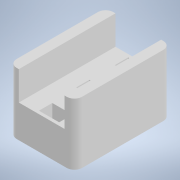
# Autodesk Inventor part: push-fit
Saved by Autodesk Inventor 2022 (Build 260153000, 153)
## iProperties
Created: 2024-10-14
Part Number: push-fit
Material: Типовые
Document SubType Name: Modeling
Designer: Andrey
Density: 1 g/cm^3
Appearance: По умолчанию
Author: Andrey
Autodesk Inventor part; units mm, degrees
ref_plane "YZ Plane" through (0, 0, 0) normal (1, 0, 0) x (0, 1, 0)
ref_plane "XZ Plane" through (0, 0, 0) normal (0, 1, 0) x (-1, 0, 0)
ref_plane "XY Plane" through (0, 0, 0) normal (0, 0, 1) x (1, 0, 0)
sketch "Эскиз1" plane through (0, 0, 0) normal (0, 1, 0) x (-1, 0, 0)
  line L0 (-2.9, 6.425) -> (2.9, 6.425)
  line L1 (2.9, 6.425) -> (2.9, -6.425)
  line L2 (2.9, -6.425) -> (-2.9, -6.425)
  line L3 (-2.9, -6.425) -> (-2.9, 6.425)
  line L4 (-2.9, 6.425) -> (2.9, -6.425) construction
  line L5 (2.9, 6.425) -> (-2.9, -6.425) construction
  line L6 (-3, 6.35) -> (3, 6.35)
  line L7 (3, 6.35) -> (3, -6.35)
  line L8 (3, -6.35) -> (-3, -6.35)
  line L9 (-3, -6.35) -> (-3, 6.35)
  line L10 (-3, 6.35) -> (3, -6.35) construction
  line L11 (3, 6.35) -> (-3, -6.35) construction
  line L12 (3, 6.35) -> (4.3, 6.35)
  line L13 (4.3, 6.35) -> (4.3, -6.35)
  line L14 (4.3, -6.35) -> (3, -6.35)
  line L15 (3, -6.35) -> (3, 6.35)
  line L16 (-3, 6.35) -> (-4.3, 6.35)
  line L17 (-4.3, 6.35) -> (-4.3, -6.35)
  line L18 (-4.3, -6.35) -> (-3, -6.35)
  line L19 (-3, -6.35) -> (-3, 6.35)
  point P0 (0, 0)
  dimension "d0" = 5.8
  dimension "d1" = 12.85
  dimension "d2" = 6
  dimension "d3" = 12.7
  dimension "d4" = 1.3
  dimension "d5" = 1.3
  constraints: 40 end point, 8 parallel, 4 horizontal, 4 midpoint, 4 perpendicular, 2 collinear
  measures "d0" distance of L1.end L2.end
  measures "d1" distance of L0.end L1.end
  measures "d2" distance of L7.end L8.end
  measures "d3" distance of L6.end L7.end
  measures "d4" distance of L13.end L14.end
  measures "d5" distance of L18.end L17.end
extrude "Выдавливание1" add sketch "Эскиз1" along normal blind 8.1 contours L6 L1 L8 L3 | L3 L8 L9 L6 | L6 L7 L8 L1 | L9 L18 L17 L16 | L12 L13 L14 L7
sketch "Эскиз2" plane through (0, 8.1, 0) normal (0, 1, 0) x (1, 0, 0)
  line L0 (4.3, 6.35) -> (-4.3, 6.35) projected
  line L1 (3, -6.35) -> (-3, -6.35)
  line L2 (-3, -6.35) -> (-3, 6.35)
  line L3 (-3, 6.35) -> (3, 6.35)
  line L4 (3, 6.35) -> (3, -6.35)
  line L5 (3, -6.35) -> (-3, 6.35) construction
  line L6 (-3, -6.35) -> (3, 6.35) construction
  point P0 (0, 0)
  dimension "d8" = 6
  constraints: 12 end point, 2 midpoint, 2 parallel, 1 horizontal, 1 perpendicular, 1 point on line
  measures "d8" distance of L2.end L3.end
extrude "Выдавливание2" cut sketch "Эскиз2" against normal blind 3.8
sketch "Эскиз3" plane through (0, 4.3, 0) normal (0, 1, 0) x (1, 0, 0)
  line L0 (3, 6.35) -> (3, -6.35) projected
  line L1 (-3, 6.35) -> (3, 6.35) projected
  line L2 (-3, -6.35) -> (-3, 6.35) projected
  line L3 (3, -6.35) -> (-3, -6.35) projected
  line L4 (3, -6.35) -> (1.7, -6.35)
  line L5 (-4.3, -6.35) -> (4.3, -6.35) projected
  line L6 (-3, -6.35) -> (-0.75, -6.35)
  line L7 (-0.75, -6.35) -> (-0.75, 6.35)
  line L8 (1.7, -6.35) -> (1.7, 6.35)
  line L9 (-3, 6.35) -> (3, 6.35) projected
  line L10 (-0.75, -6.35) -> (1.7, -6.35)
  line L11 (0.475, -6.35) -> (0.475, 6.35)
  line L12 (0.475, -5.08) -> (0.475, 0)
  line L13 (0.475, 0) -> (0.475, 5.08)
  line L14 (1.7, 0) -> (-0.75, 0)
  line L15 (-0.75, -0.675) -> (1.7, -0.675)
  line L16 (1.7, -0.675) -> (1.7, 0.675)
  line L17 (1.7, 0.675) -> (-0.75, 0.675)
  line L18 (-0.75, 0.675) -> (-0.75, -0.675)
  line L19 (-0.75, -0.675) -> (1.7, 0.675) construction
  line L20 (1.7, -0.675) -> (-0.75, 0.675) construction
  line L21 (-0.75, 4.405) -> (1.7, 4.405)
  line L22 (1.7, 4.405) -> (1.7, 5.755)
  line L23 (1.7, 5.755) -> (-0.75, 5.755)
  line L24 (-0.75, 5.755) -> (-0.75, 4.405)
  line L25 (-0.75, 4.405) -> (1.7, 5.755) construction
  line L26 (1.7, 4.405) -> (-0.75, 5.755) construction
  line L27 (-0.75, -5.755) -> (1.7, -5.755)
  line L28 (1.7, -5.755) -> (1.7, -4.405)
  line L29 (1.7, -4.405) -> (-0.75, -4.405)
  line L30 (-0.75, -4.405) -> (-0.75, -5.755)
  line L31 (-0.75, -5.755) -> (1.7, -4.405) construction
  line L32 (1.7, -5.755) -> (-0.75, -4.405) construction
  line L33 (-0.95, 0.875) -> (1.9, 0.875)
  line L34 (1.9, 0.875) -> (1.9, -0.875)
  line L35 (1.9, -0.875) -> (-0.95, -0.875)
  line L36 (-0.95, -0.875) -> (-0.95, 0.875)
  line L37 (1.9, 4.205) -> (-0.95, 4.205)
  line L38 (-0.95, 4.205) -> (-0.95, 5.955)
  line L39 (-0.95, 5.955) -> (1.9, 5.955)
  line L40 (1.9, 5.955) -> (1.9, 4.205)
  line L41 (-0.95, -4.205) -> (1.9, -4.205)
  line L42 (1.9, -4.205) -> (1.9, -5.955)
  line L43 (1.9, -5.955) -> (-0.95, -5.955)
  line L44 (-0.95, -5.955) -> (-0.95, -4.205)
  line L45 (-0.95, 5.955) -> (1.9, 5.955)
  line L46 (1.9, 5.955) -> (1.9, 4.205)
  line L47 (1.9, 4.205) -> (-0.95, 4.205)
  line L48 (-0.95, 4.205) -> (-0.95, 5.955)
  point P0 (0, 0)
  point P1 (-0.75, -4.205)
  point P2 (-0.75, -5.955)
  point P3 (-0.75, 4.205)
  point P4 (-0.75, 5.955)
  point P5 (-0.75, 5.955)
  dimension "d11" = 1.3
  dimension "d12" = 2.25
  dimension "d13" = 5.08
  dimension "d14" = 5.08
  dimension "d15" = 1.35
  dimension "d16" = 1.35
  dimension "d17" = 1.35
  dimension "d18" = 0.2
  dimension "d19" = 0.2
  dimension "d20" = 0.2
  constraints: 86 end point, 14 parallel, 10 midpoint, 10 point on line, 9 perpendicular, 4 horizontal, 1 collinear, 1 vertical, 9 other
  measures "d11" distance of L0.end L4.end
  measures "d12" distance of L2.start L6.end
  measures "d13" distance of L12.end L12.start
  measures "d14" distance of L12.end L13.end
  measures "d15" distance of L16.end L15.end
  measures "d16" distance of L22.end L21.end
  measures "d17" distance of L28.end L27.end
  measures "d18" distance between parallel lines of L17 L33
  measures "d19" distance between parallel lines of L21 L37
  measures "d20" distance between parallel lines of L29 L41
extrude "Выдавливание3" cut sketch "Эскиз3" against normal blind 4 contours L39 L40 L37 L8 | L8 L23 L11 L39 | L43 L11 L27 L8 | L8 L41 L42 L43 | L11 L23 L7 L39 | L8 L21 L11 L23 | L43 L7 L27 L11 | L27 L11 L29 L8 | L7 L37 L38 L39 | L11 L21 L7 L23 | L8 L37 L11 L21 | L27 L7 L29 L11 | L29 L11 L41 L8 | L11 L37 L7 L21 | L29 L7 L41 L11 | L33 L34 L35 L8 | L8 L17 L11 L33 | L35 L11 L15 L8 | L8 L14 L11 L17 | L11 L17 L7 L33 | L15 L11 L14 L8 | L35 L7 L15 L11 | L7 L35 L36 L33 | L11 L14 L7 L17 | L15 L7 L14 L11
sketch "Эскиз4" plane through (0, 0.3, 0) normal (0, 1, 0) x (1, 0, 0)
  line L0 (1.9, -5.955) -> (-0.75, -5.955) projected
  line L1 (-0.75, -5.955) -> (-0.75, -4.205) projected
  line L2 (-0.75, -4.205) -> (1.9, -4.205) projected
  line L3 (1.9, -4.205) -> (1.9, -5.955) projected
  line L4 (1.9, 5.955) -> (1.9, 4.205) projected
  line L5 (1.9, 4.205) -> (-0.95, 4.205) projected
  line L6 (-0.95, 4.205) -> (-0.95, 5.955) projected
  line L7 (-0.95, 5.955) -> (1.9, 5.955) projected
  line L8 (1.9, -0.875) -> (-0.95, -0.875) projected
  line L9 (-0.95, -0.875) -> (-0.95, 0.875) projected
  line L10 (-0.95, 0.875) -> (1.9, 0.875) projected
  line L11 (1.9, 0.875) -> (1.9, -0.875) projected
  line L12 (3, 6.35) -> (3, -6.35) projected
  line L13 (-3, 6.35) -> (3, 6.35) projected
  line L14 (-3, -6.35) -> (-3, 6.35) projected
  line L15 (3, -6.35) -> (-3, -6.35) projected
  line L16 (0, -0.875) -> (-0.4, -0.875)
  line L17 (-0.4, -0.875) -> (-0.4, 0.875)
  line L18 (-0.4, 0.875) -> (0, 0.875)
  line L19 (0, 0.875) -> (0, -0.875)
  line L20 (1.9, 4.205) -> (-0.95, 4.205) projected
  line L21 (0, 4.205) -> (-0.4, 4.205)
  line L22 (-0.4, 4.205) -> (-0.4, 5.955)
  line L23 (-0.4, 5.955) -> (0, 5.955)
  line L24 (0, 5.955) -> (0, 4.205)
  line L25 (1.9, -5.955) -> (-0.75, -5.955) projected
  line L26 (-0.75, -4.205) -> (1.9, -4.205) projected
  line L27 (0, -5.955) -> (-0.4, -5.955)
  line L28 (-0.4, -5.955) -> (-0.4, -4.205)
  line L29 (-0.4, -4.205) -> (0, -4.205)
  line L30 (0, -4.205) -> (0, -5.955)
  line L31 (3, -6.35) -> (-3, -6.35) projected
  line L32 (0, -6.35) -> (0, 6.35)
  line L33 (4.3, 6.35) -> (-4.3, 6.35) projected
  point P0 (0, 0)
  dimension "d23" = 0.4
  constraints: 26 end point, 9 point on line, 6 parallel, 3 horizontal, 3 perpendicular, 2 collinear, 2 midpoint
  measures "d23" distance between parallel lines of L32 L22
extrude "Выдавливание4" cut sketch "Эскиз4" against normal blind 4 contours L0 L28 L2 L30 | L8 L17 L10 L19 | L5 L22 L7 L24
fillet "Сопряжение1" radius 1 4 edges at (4.3, 4.05, 6.35) (-4.3, 4.05, 6.35) (-4.3, 4.05, -6.35) (4.3, 4.05, -6.35)
